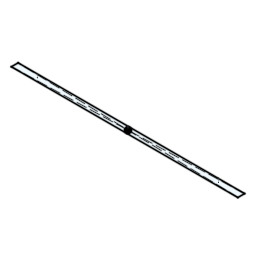
Template (Autodesk Fusion 360 design; units mm, degrees)
Autodesk Fusion 360 part; units mm, degrees
sketch "Contact Area" plane through (0, 0, 0) normal (0, 0, 1) x (1, 0, 0)
  line L0 (300, -9) -> (-300, -9)
  line L1 (-300, -9) -> (-300, 9)
  line L2 (-300, 9) -> (300, 9)
  line L3 (300, 9) -> (300, -9)
  line L4 (300, -9) -> (-300, 9) construction
  line L5 (-300, -9) -> (300, 9) construction
  dimension "d3" = 600
  dimension "d4" = 18
  constraint horizontal L0
  constraint perpendicular L0 L1
  constraint parallel L0 L2
  constraint parallel L1 L3
  constraint coincident L4 origin
  constraint coincident L5 origin
  measures "d3" distance of L0.start L0.end
  measures "d4" distance of L0 L2
sketch "Pins" plane through (0, 0, 0) normal (0, 0, 1) x (1, 0, 0)
  circle A0 centre (240, 0) radius 0.5
  line L0 (300, 9) -> (300, -9)
  line L1 (-300, 9) -> (300, 9)
  circle A1 centre (-240, 0) radius 0.5
  line L2 (-300, -9) -> (-300, 9)
  dimension "d8" = 1
  dimension "d9" = 60
  dimension "d10" = 9
  dimension "d11" = 1
  dimension "d12" = 60
  dimension "d13" = 9
  measures "d8" diameter of A0
  measures "d9" distance of A0.centre L0
  measures "d10" distance of A0.centre L1
  measures "d11" diameter of A1
  measures "d12" distance of A1.centre L2
  measures "d13" distance of L1 A1.centre
extrude "Extrude1" add sketch "Pins" along normal blind 10 contours A0 makes body 1
pattern_linear "R-Pattern1" count 3 spacing 240 along (-1, 0, 0) of bodies 1 makes body 2 at (0.4994, -0.0249, 6.6667) makes body 3 at (-240.383, 0.3214, 6.6667)
equation "ContactAreaLength = 600 mm" comment "Length of the a contact area, calculated automatically"
equation "ContactAreaWidth = 18 mm" comment "Width of a contact area. Calculated automatically"
equation "d3 = ContactAreaLength"
equation "d4 = ContactAreaWidth"
equation "UserOffset1 = 60 mm" comment "Offset from the edge"
equation "UserOffset2 = 60 mm" comment "Offset from the edge"
equation "CoordY = ContactAreaWidth / 2"
equation "d9 = UserOffset1"
equation "d10 = CoordY"
equation "d12 = Offset2"
equation "d13 = CoordY"
equation "MaxDistance = 300 mm" comment "Max distance between components"
equation "MinDistance = 32 mm" comment "Min distance between components"
equation "Offset1 = if(PlacingLength >= MinDistance; UserOffset1; ContactAreaLength / 2)"
equation "Offset2 = if(PlacingLength >= MinDistance; UserOffset2; Offset1)"
equation "PlacingLength = ContactAreaLength - UserOffset1 - UserOffset2" comment "Space between components"
equation "NumberOfIntervals = ceil(PlacingLength / MaxDistance)" comment "Number of intervals between components"
equation "NumberOfComponents = if(PlacingLength >= MinDistance; NumberOfIntervals + 1; 1)" comment "Number of components, calculated automatically"
equation "SpaceBetween = if(PlacingLength >= MinDistance; PlacingLength / NumberOfIntervals; 0 mm)" comment "Space between components"
equation "d27 = NumberOfComponents"
equation "d29 = SpaceBetween"
named bodies: "Pin1", "Pin1 (1)", "Pin1 (2)"
